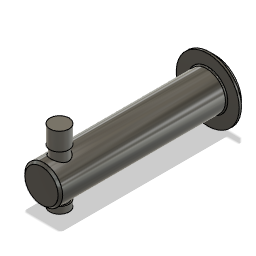
0.175.7657 - Axe d'articulation avec tête 8,40 type B + Goupille fendue 2x14-A (Autodesk Fusion 360 design; units mm, degrees)
Autodesk Fusion 360 part; units mm, degrees
sketch "Sketch1" plane through (0, 0, 0) normal (0, 0, 1) x (1, 0, 0)
  circle A0 centre (0, 0) radius 4.2
  dimension "d1" = 8.4
  constraint coincident A0.centre origin
  measures "d1" diameter of A0
extrude "Extrude1" add sketch "Sketch1" along normal blind 37 makes body 1
sketch "Sketch2" plane through (0, 0, 0) normal (0, 0, -1) x (-1, 0, 0)
  circle A0 centre (0, 0) radius 4.2
  circle A1 centre (0, 0) radius 7
  dimension "d4" = 14
  constraint coincident A0.centre A1.centre
  measures "d4" diameter of A1
extrude "Extrude2" add sketch "Sketch2" along normal blind 1.5 contours A0 | A1 bodies 1
chamfer "Chamfer1" distance 1 angle 45 1 edges at (6.5263, -2.5313, -1.5) on bodies 1
sketch "Sketch3" plane through (0, 0, 0) normal (0, 1, 0) x (1, 0, 0)
  line L0 (7, 0) -> (-7, 0)
  line L1 (-4.2, 0) -> (18, 0) construction
  line L2 (-4.2, -20) -> (18, -20) construction
  line L3 (0, 0) -> (0, -20) construction
  line L4 (0, -20) -> (0, -33) construction
  circle A0 centre (0, -33) radius 2
  point P0 (-4.2, 0)
  dimension "d8" = 20
  dimension "d9" = 4
  dimension "d24" = 13
  constraint coincident P0 L1.start
  constraint parallel L0 L1
  constraint coincident L3.start origin
  constraint coincident L2 L3.end
  constraint perpendicular L2 L3
  constraint perpendicular L2 L4
  constraint coincident L4.end A0.centre
  measures "d9" diameter of A0
  measures "d24" vertical distance of L3.end L4.end
extrude "Extrude3" cut sketch "Sketch3" along normal through all and the other way through all bodies 1
sketch "Sketch4" plane through (0, 0, 0) normal (0, 1, 0) x (1, 0, 0)
  circle A0 centre (0, -33) radius 1.8028
extrude "Extrude4" add sketch "Sketch4" along normal blind 10 and the other way blind 6 separate body makes body 2
sketch "Sketch5" plane through (0, -6, 0) normal (0, -1, 0) x (1, 0, 0)
  circle A0 centre (0, 33) radius 1.8028
  circle A1 centre (0, 33) radius 2.125
  dimension "d21" = 4.25
  constraint concentric A0 A1
  measures "d21" diameter of A1
extrude "Extrude5" add sketch "Sketch5" against normal blind 1.5 contours A0 | A1 bodies 2
sketch "Sketch6" plane through (0, 10, 0) normal (0, 1, 0) x (-1, 0, 0)
  circle A0 centre (0, 33) radius 1.8028
  circle A1 centre (0, 33) radius 2.125
  circle A2 centre (0, 33) radius 2.125
  circle A3 centre (0, 33) radius 2.125
  dimension "d20" = 4.25
  constraint concentric A0 A1
  measures "d20" diameter of A1
extrude "Extrude6" add sketch "Sketch6" against normal blind 4 bodies 2
chamfer "Chamfer2" distance 0.5 angle 45 1 edges at (-3.9158, -1.5188, 37) on bodies 1
fillet "Fillet1" radius 0.25 1 edges at (-3.9158, -1.5188, 0) on bodies 1
